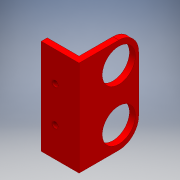
# Autodesk Inventor part: Part1
Saved by Autodesk Inventor 2017 (Build 210142000, 142)
## iProperties
Created: 2017-12-21
Part Number: Part1
Material: Generic
Document SubType Name: Modeling
Designer: Dharsan
Density: 1 g/cm^3
Appearance: Default
Author: Dharsan
Autodesk Inventor part; units mm, degrees
ref_plane "YZ Plane" through (0, 0, 0) normal (1, 0, 0) x (0, 1, 0)
ref_plane "XZ Plane" through (0, 0, 0) normal (0, 1, 0) x (-1, 0, 0)
ref_plane "XY Plane" through (0, 0, 0) normal (0, 0, 1) x (1, 0, 0)
sketch "Sketch1" plane through (0, 0, 0) normal (0, 0, 1) x (1, 0, 0)
  line L0 (0, 0) -> (0, 3)
  line L1 (0, 3) -> (16, 3)
  line L2 (0, 0) -> (19, 0)
  line L3 (19, 0) -> (19, 30)
  line L4 (16, 3) -> (16, 30)
  line L5 (16, 30) -> (19, 30)
  dimension "d0" = 3
  dimension "d1" = 16
  dimension "d2" = 19
  dimension "d3" = 30
  constraints: 12 end point, 3 perpendicular, 2 vertical, 1 horizontal
  measures "d0" distance of L0.start L0.end
  measures "d1" distance of L0.end L1.end
  measures "d2" distance of L0.start L2.end
  measures "d3" distance of L2.end L3.end
extrude "Extrusion1" add sketch "Sketch1" along normal blind 48
fillet "Fillet1" radius 10 2 edges at (17.5, 30, 0) (17.5, 30, 48)
sketch "Sketch2" plane through (19, 0, 48) normal (1, 0, 0) x (0, 0, -1)
  circle A0 centre (11, 20) radius 8.35
  circle A1 centre (37, 20) radius 8.35
  line L0 (48, 20) -> (48, 0) projected
  line L1 (38, 30) -> (10, 30) projected
  line L2 (0, 0) -> (0, 20) projected
  dimension "d7" = 16.7
  dimension "d8" = 16.7
  dimension "d9" = 11
  dimension "d10" = 10
  dimension "d11" = 10
  dimension "d12" = 11
  constraints: 2 centre point
  measures "d7" diameter of A0
  measures "d8" diameter of A1
  measures "d9" distance from line of L0 A1.centre
  measures "d10" distance from line of L1 A1.centre
  measures "d11" distance from line of L1 A0.centre
  measures "d12" distance from line of L2 A0.centre
extrude "Extrusion2" cut sketch "Sketch2" against normal blind 48
sketch "Sketch3" plane through (0, 3, 0) normal (0, 1, 0) x (1, 0, 0)
  circle A0 centre (7, -33) radius 1.5
  circle A1 centre (7, -15) radius 1.5
  line L0 (0, 0) -> (16, 0) projected
  line L1 (16, -48) -> (0, -48) projected
  line L2 (0, 0) -> (0, -48) projected
  dimension "d15" = 3
  dimension "d16" = 3
  dimension "d17" = 15
  dimension "d18" = 15
  dimension "d19" = 7
  dimension "d20" = 7
  constraints: 2 centre point
  measures "d15" diameter of A0
  measures "d16" diameter of A1
  measures "d17" distance from line of L0 A1.centre
  measures "d18" distance from line of L1 A0.centre
  measures "d19" distance from line of L2 A0.centre
  measures "d20" distance from line of L2 A1.centre
extrude "Extrusion3" cut sketch "Sketch3" against normal blind 48
body "Solid1"
